Autodesk Inventor part; units mm, degrees
(part 2 of 13)
  line L395 (2.337, 43.029) -> (2.4628, 43.029)
  arc A395 (2.4628, 43.029) -> (2.4628, 43.155) centre (2.4628, 43.092) ccw
  line L396 (2.4628, 43.155) -> (2.337, 43.155)
  arc A396 (2.337, 43.155) -> (2.337, 43.029) centre (2.337, 43.092) ccw
  line L397 (3.263, 43.029) -> (17.121, 43.029)
  arc A397 (17.121, 43.029) -> (17.121, 43.155) centre (17.121, 43.092) ccw
  line L398 (17.121, 43.155) -> (3.263, 43.155)
  arc A398 (3.263, 43.155) -> (3.263, 43.029) centre (3.263, 43.092) ccw
  line L399 (1.0789, 43.155) -> (1.4109, 43.155)
  arc A399 (1.4109, 43.155) -> (1.4109, 43.281) centre (1.4109, 43.218) ccw
  line L400 (1.4109, 43.281) -> (1.0789, 43.281)
  arc A400 (1.0789, 43.281) -> (1.0789, 43.155) centre (1.0789, 43.218) ccw
  line L401 (2.337, 43.155) -> (2.4628, 43.155)
  arc A401 (2.4628, 43.155) -> (2.4628, 43.281) centre (2.4628, 43.218) ccw
  line L402 (2.4628, 43.281) -> (2.337, 43.281)
  arc A402 (2.337, 43.281) -> (2.337, 43.155) centre (2.337, 43.218) ccw
  line L403 (3.389, 43.155) -> (17.121, 43.155)
  arc A403 (17.121, 43.155) -> (17.121, 43.281) centre (17.121, 43.218) ccw
  line L404 (17.121, 43.281) -> (3.389, 43.281)
  arc A404 (3.389, 43.281) -> (3.389, 43.155) centre (3.389, 43.218) ccw
  line L405 (1.0789, 43.281) -> (1.3337, 43.281)
  arc A405 (1.3337, 43.281) -> (1.3337, 43.407) centre (1.3337, 43.344) ccw
  line L406 (1.3337, 43.407) -> (1.0789, 43.407)
  arc A406 (1.0789, 43.407) -> (1.0789, 43.281) centre (1.0789, 43.344) ccw
  line L407 (2.337, 43.281) -> (2.4628, 43.281)
  arc A407 (2.4628, 43.281) -> (2.4628, 43.407) centre (2.4628, 43.344) ccw
  line L408 (2.4628, 43.407) -> (2.337, 43.407)
  arc A408 (2.337, 43.407) -> (2.337, 43.281) centre (2.337, 43.344) ccw
  line L409 (3.4661, 43.281) -> (17.121, 43.281)
  arc A409 (17.121, 43.281) -> (17.121, 43.407) centre (17.121, 43.344) ccw
  line L410 (17.121, 43.407) -> (3.4661, 43.407)
  arc A410 (3.4661, 43.407) -> (3.4661, 43.281) centre (3.4661, 43.344) ccw
  line L411 (1.0789, 43.407) -> (1.2815, 43.407)
  arc A411 (1.2815, 43.407) -> (1.2815, 43.533) centre (1.2815, 43.47) ccw
  line L412 (1.2815, 43.533) -> (1.0789, 43.533)
  arc A412 (1.0789, 43.533) -> (1.0789, 43.407) centre (1.0789, 43.47) ccw
  line L413 (2.337, 43.407) -> (2.4628, 43.407)
  arc A413 (2.4628, 43.407) -> (2.4628, 43.533) centre (2.4628, 43.47) ccw
  line L414 (2.4628, 43.533) -> (2.337, 43.533)
  arc A414 (2.337, 43.533) -> (2.337, 43.407) centre (2.337, 43.47) ccw
  line L415 (3.5183, 43.407) -> (7.3627, 43.407)
  arc A415 (7.3627, 43.407) -> (7.3627, 43.533) centre (7.3627, 43.47) ccw
  line L416 (7.3627, 43.533) -> (3.5183, 43.533)
  arc A416 (3.5183, 43.533) -> (3.5183, 43.407) centre (3.5183, 43.47) ccw
  line L417 (8.0371, 43.407) -> (17.121, 43.407)
  arc A417 (17.121, 43.407) -> (17.121, 43.533) centre (17.121, 43.47) ccw
  line L418 (17.121, 43.533) -> (8.0371, 43.533)
  arc A418 (8.0371, 43.533) -> (8.0371, 43.407) centre (8.0371, 43.47) ccw
  line L419 (1.0789, 43.533) -> (1.2293, 43.533)
  arc A419 (1.2293, 43.533) -> (1.2293, 43.659) centre (1.2293, 43.596) ccw
  line L420 (1.2293, 43.659) -> (1.0789, 43.659)
  arc A420 (1.0789, 43.659) -> (1.0789, 43.533) centre (1.0789, 43.596) ccw
  line L421 (2.337, 43.533) -> (2.4628, 43.533)
  arc A421 (2.4628, 43.533) -> (2.4628, 43.659) centre (2.4628, 43.596) ccw
  line L422 (2.4628, 43.659) -> (2.337, 43.659)
  arc A422 (2.337, 43.659) -> (2.337, 43.533) centre (2.337, 43.596) ccw
  line L423 (3.5705, 43.533) -> (7.0585, 43.533)
  arc A423 (7.0585, 43.533) -> (7.0585, 43.659) centre (7.0585, 43.596) ccw
  line L424 (7.0585, 43.659) -> (3.5705, 43.659)
  arc A424 (3.5705, 43.659) -> (3.5705, 43.533) centre (3.5705, 43.596) ccw
  line L425 (8.3413, 43.533) -> (17.121, 43.533)
  arc A425 (17.121, 43.533) -> (17.121, 43.659) centre (17.121, 43.596) ccw
  line L426 (17.121, 43.659) -> (8.3413, 43.659)
  arc A426 (8.3413, 43.659) -> (8.3413, 43.533) centre (8.3413, 43.596) ccw
  line L427 (1.0789, 43.659) -> (1.183, 43.659)
  arc A427 (1.183, 43.659) -> (1.183, 43.785) centre (1.183, 43.722) ccw
  line L428 (1.183, 43.785) -> (1.0789, 43.785)
  arc A428 (1.0789, 43.785) -> (1.0789, 43.659) centre (1.0789, 43.722) ccw
  line L429 (2.337, 43.659) -> (2.4628, 43.659)
  arc A429 (2.4628, 43.659) -> (2.4628, 43.785) centre (2.4628, 43.722) ccw
  line L430 (2.4628, 43.785) -> (2.337, 43.785)
  arc A430 (2.337, 43.785) -> (2.337, 43.659) centre (2.337, 43.722) ccw
  line L431 (3.6169, 43.659) -> (6.8884, 43.659)
  arc A431 (6.8884, 43.659) -> (6.8884, 43.785) centre (6.8884, 43.722) ccw
  line L432 (6.8884, 43.785) -> (3.6169, 43.785)
  arc A432 (3.6169, 43.785) -> (3.6169, 43.659) centre (3.6169, 43.722) ccw
  line L433 (8.5115, 43.659) -> (17.121, 43.659)
  arc A433 (17.121, 43.659) -> (17.121, 43.785) centre (17.121, 43.722) ccw
  line L434 (17.121, 43.785) -> (8.5115, 43.785)
  arc A434 (8.5115, 43.785) -> (8.5115, 43.659) centre (8.5115, 43.722) ccw
  line L435 (1.0789, 43.785) -> (1.183, 43.785)
  arc A435 (1.183, 43.785) -> (1.183, 43.911) centre (1.183, 43.848) ccw
  line L436 (1.183, 43.911) -> (1.0789, 43.911)
  arc A436 (1.0789, 43.911) -> (1.0789, 43.785) centre (1.0789, 43.848) ccw
  line L437 (2.337, 43.785) -> (2.4628, 43.785)
  arc A437 (2.4628, 43.785) -> (2.4628, 43.911) centre (2.4628, 43.848) ccw
  line L438 (2.4628, 43.911) -> (2.337, 43.911)
  arc A438 (2.337, 43.911) -> (2.337, 43.785) centre (2.337, 43.848) ccw
  line L439 (3.6169, 43.785) -> (6.7624, 43.785)
  arc A439 (6.7624, 43.785) -> (6.7624, 43.911) centre (6.7624, 43.848) ccw
  line L440 (6.7624, 43.911) -> (3.6169, 43.911)
  arc A440 (3.6169, 43.911) -> (3.6169, 43.785) centre (3.6169, 43.848) ccw
  line L441 (8.6375, 43.785) -> (17.121, 43.785)
  arc A441 (17.121, 43.785) -> (17.121, 43.911) centre (17.121, 43.848) ccw
  line L442 (17.121, 43.911) -> (8.6375, 43.911)
  arc A442 (8.6375, 43.911) -> (8.6375, 43.785) centre (8.6375, 43.848) ccw
  line L443 (1.0789, 43.911) -> (2.3365, 43.911)
  arc A443 (2.3365, 43.911) -> (2.3365, 44.037) centre (2.3365, 43.974) ccw
  line L444 (2.3365, 44.037) -> (1.0789, 44.037)
  arc A444 (1.0789, 44.037) -> (1.0789, 43.911) centre (1.0789, 43.974) ccw
  line L445 (2.4634, 43.911) -> (6.6364, 43.911)
  arc A445 (6.6364, 43.911) -> (6.6364, 44.037) centre (6.6364, 43.974) ccw
  line L446 (6.6364, 44.037) -> (2.4634, 44.037)
  arc A446 (2.4634, 44.037) -> (2.4634, 43.911) centre (2.4634, 43.974) ccw
  line L447 (8.7635, 43.911) -> (17.121, 43.911)
  arc A447 (17.121, 43.911) -> (17.121, 44.037) centre (17.121, 43.974) ccw
  line L448 (17.121, 44.037) -> (8.7635, 44.037)
  arc A448 (8.7635, 44.037) -> (8.7635, 43.911) centre (8.7635, 43.974) ccw
  line L449 (1.0789, 44.037) -> (1.183, 44.037)
  arc A449 (1.183, 44.037) -> (1.183, 44.163) centre (1.183, 44.1) ccw
  line L450 (1.183, 44.163) -> (1.0789, 44.163)
  arc A450 (1.0789, 44.163) -> (1.0789, 44.037) centre (1.0789, 44.1) ccw
  line L451 (2.337, 44.037) -> (2.4628, 44.037)
  arc A451 (2.4628, 44.037) -> (2.4628, 44.163) centre (2.4628, 44.1) ccw
  line L452 (2.4628, 44.163) -> (2.337, 44.163)
  arc A452 (2.337, 44.163) -> (2.337, 44.037) centre (2.337, 44.1) ccw
  line L453 (3.6169, 44.037) -> (6.5788, 44.037)
  arc A453 (6.5788, 44.037) -> (6.5788, 44.163) centre (6.5788, 44.1) ccw
  line L454 (6.5788, 44.163) -> (3.6169, 44.163)
  arc A454 (3.6169, 44.163) -> (3.6169, 44.037) centre (3.6169, 44.1) ccw
  line L455 (8.821, 44.037) -> (17.121, 44.037)
  arc A455 (17.121, 44.037) -> (17.121, 44.163) centre (17.121, 44.1) ccw
  line L456 (17.121, 44.163) -> (8.821, 44.163)
  arc A456 (8.821, 44.163) -> (8.821, 44.037) centre (8.821, 44.1) ccw
  line L457 (1.0789, 44.163) -> (1.1971, 44.163)
  arc A457 (1.1971, 44.163) -> (1.1971, 44.289) centre (1.1971, 44.226) ccw
  line L458 (1.1971, 44.289) -> (1.0789, 44.289)
  arc A458 (1.0789, 44.289) -> (1.0789, 44.163) centre (1.0789, 44.226) ccw
  line L459 (2.337, 44.163) -> (2.4628, 44.163)
  arc A459 (2.4628, 44.163) -> (2.4628, 44.289) centre (2.4628, 44.226) ccw
  line L460 (2.4628, 44.289) -> (2.337, 44.289)
  arc A460 (2.337, 44.289) -> (2.337, 44.163) centre (2.337, 44.226) ccw
  line L461 (3.6029, 44.163) -> (6.5266, 44.163)
  arc A461 (6.5266, 44.163) -> (6.5266, 44.289) centre (6.5266, 44.226) ccw
  line L462 (6.5266, 44.289) -> (3.6029, 44.289)
  arc A462 (3.6029, 44.289) -> (3.6029, 44.163) centre (3.6029, 44.226) ccw
  line L463 (8.8732, 44.163) -> (17.121, 44.163)
  arc A463 (17.121, 44.163) -> (17.121, 44.289) centre (17.121, 44.226) ccw
  line L464 (17.121, 44.289) -> (8.8732, 44.289)
  arc A464 (8.8732, 44.289) -> (8.8732, 44.163) centre (8.8732, 44.226) ccw
  line L465 (1.0789, 44.289) -> (1.2493, 44.289)
  arc A465 (1.2493, 44.289) -> (1.2493, 44.415) centre (1.2493, 44.352) ccw
  line L466 (1.2493, 44.415) -> (1.0789, 44.415)
  arc A466 (1.0789, 44.415) -> (1.0789, 44.289) centre (1.0789, 44.352) ccw
  line L467 (2.337, 44.289) -> (2.4628, 44.289)
  arc A467 (2.4628, 44.289) -> (2.4628, 44.415) centre (2.4628, 44.352) ccw
  line L468 (2.4628, 44.415) -> (2.337, 44.415)
  arc A468 (2.337, 44.415) -> (2.337, 44.289) centre (2.337, 44.352) ccw
  line L469 (3.5507, 44.289) -> (6.4744, 44.289)
  arc A469 (6.4744, 44.289) -> (6.4744, 44.415) centre (6.4744, 44.352) ccw
  line L470 (6.4744, 44.415) -> (3.5507, 44.415)
  arc A470 (3.5507, 44.415) -> (3.5507, 44.289) centre (3.5507, 44.352) ccw
  line L471 (8.9254, 44.289) -> (17.121, 44.289)
  arc A471 (17.121, 44.289) -> (17.121, 44.415) centre (17.121, 44.352) ccw
  line L472 (17.121, 44.415) -> (8.9254, 44.415)
  arc A472 (8.9254, 44.415) -> (8.9254, 44.289) centre (8.9254, 44.352) ccw
  line L473 (1.0789, 44.415) -> (1.3015, 44.415)
  arc A473 (1.3015, 44.415) -> (1.3015, 44.541) centre (1.3015, 44.478) ccw
  line L474 (1.3015, 44.541) -> (1.0789, 44.541)
  arc A474 (1.0789, 44.541) -> (1.0789, 44.415) centre (1.0789, 44.478) ccw
  line L475 (2.337, 44.415) -> (2.4628, 44.415)
  arc A475 (2.4628, 44.415) -> (2.4628, 44.541) centre (2.4628, 44.478) ccw
  line L476 (2.4628, 44.541) -> (2.337, 44.541)
  arc A476 (2.337, 44.541) -> (2.337, 44.415) centre (2.337, 44.478) ccw
  line L477 (3.4985, 44.415) -> (6.4346, 44.415)
  arc A477 (6.4346, 44.415) -> (6.4346, 44.541) centre (6.4346, 44.478) ccw
  line L478 (6.4346, 44.541) -> (3.4985, 44.541)
  arc A478 (3.4985, 44.541) -> (3.4985, 44.415) centre (3.4985, 44.478) ccw
  line L479 (8.9653, 44.415) -> (17.121, 44.415)
  arc A479 (17.121, 44.415) -> (17.121, 44.541) centre (17.121, 44.478) ccw
  line L480 (17.121, 44.541) -> (8.9653, 44.541)
  arc A480 (8.9653, 44.541) -> (8.9653, 44.415) centre (8.9653, 44.478) ccw
  line L481 (1.0789, 44.541) -> (1.3537, 44.541)
  arc A481 (1.3537, 44.541) -> (1.3537, 44.667) centre (1.3537, 44.604) ccw
  line L482 (1.3537, 44.667) -> (1.0789, 44.667)
  arc A482 (1.0789, 44.667) -> (1.0789, 44.541) centre (1.0789, 44.604) ccw
  line L483 (2.337, 44.541) -> (2.4628, 44.541)
  arc A483 (2.4628, 44.541) -> (2.4628, 44.667) centre (2.4628, 44.604) ccw
  line L484 (2.4628, 44.667) -> (2.337, 44.667)
  arc A484 (2.337, 44.667) -> (2.337, 44.541) centre (2.337, 44.604) ccw
  line L485 (3.4463, 44.541) -> (6.4346, 44.541)
  arc A485 (6.4346, 44.541) -> (6.4346, 44.667) centre (6.4346, 44.604) ccw
  line L486 (6.4346, 44.667) -> (3.4463, 44.667)
  arc A486 (3.4463, 44.667) -> (3.4463, 44.541) centre (3.4463, 44.604) ccw
  line L487 (8.9653, 44.541) -> (17.121, 44.541)
  arc A487 (17.121, 44.541) -> (17.121, 44.667) centre (17.121, 44.604) ccw
  line L488 (17.121, 44.667) -> (8.9653, 44.667)
  arc A488 (8.9653, 44.667) -> (8.9653, 44.541) centre (8.9653, 44.604) ccw
  line L489 (1.0789, 44.667) -> (1.459, 44.667)
  arc A489 (1.459, 44.667) -> (1.459, 44.793) centre (1.459, 44.73) ccw
  line L490 (1.459, 44.793) -> (1.0789, 44.793)
  arc A490 (1.0789, 44.793) -> (1.0789, 44.667) centre (1.0789, 44.73) ccw
  line L491 (2.337, 44.667) -> (2.4628, 44.667)
  arc A491 (2.4628, 44.667) -> (2.4628, 44.793) centre (2.4628, 44.73) ccw
  line L492 (2.4628, 44.793) -> (2.337, 44.793)
  arc A492 (2.337, 44.793) -> (2.337, 44.667) centre (2.337, 44.73) ccw
  line L493 (3.3409, 44.667) -> (6.4346, 44.667)
  arc A493 (6.4346, 44.667) -> (6.4346, 44.793) centre (6.4346, 44.73) ccw
  line L494 (6.4346, 44.793) -> (3.3409, 44.793)
  arc A494 (3.3409, 44.793) -> (3.3409, 44.667) centre (3.3409, 44.73) ccw
  line L495 (8.9653, 44.667) -> (17.121, 44.667)
  arc A495 (17.121, 44.667) -> (17.121, 44.793) centre (17.121, 44.73) ccw
  line L496 (17.121, 44.793) -> (8.9653, 44.793)
  arc A496 (8.9653, 44.793) -> (8.9653, 44.667) centre (8.9653, 44.73) ccw
  line L497 (1.0789, 44.793) -> (1.585, 44.793)
  arc A497 (1.585, 44.793) -> (1.585, 44.919) centre (1.585, 44.856) ccw
  line L498 (1.585, 44.919) -> (1.0789, 44.919)
  arc A498 (1.0789, 44.919) -> (1.0789, 44.793) centre (1.0789, 44.856) ccw
  line L499 (2.337, 44.793) -> (2.4628, 44.793)
  arc A499 (2.4628, 44.793) -> (2.4628, 44.919) centre (2.4628, 44.856) ccw
  line L500 (2.4628, 44.919) -> (2.337, 44.919)
  arc A500 (2.337, 44.919) -> (2.337, 44.793) centre (2.337, 44.856) ccw
  line L501 (3.2149, 44.793) -> (6.4346, 44.793)
  arc A501 (6.4346, 44.793) -> (6.4346, 44.919) centre (6.4346, 44.856) ccw
  line L502 (6.4346, 44.919) -> (3.2149, 44.919)
  arc A502 (3.2149, 44.919) -> (3.2149, 44.793) centre (3.2149, 44.856) ccw
  line L503 (8.9653, 44.793) -> (17.121, 44.793)
  arc A503 (17.121, 44.793) -> (17.121, 44.919) centre (17.121, 44.856) ccw
  line L504 (17.121, 44.919) -> (8.9653, 44.919)
  arc A504 (8.9653, 44.919) -> (8.9653, 44.793) centre (8.9653, 44.856) ccw
  line L505 (1.0789, 44.919) -> (1.7116, 44.919)
  arc A505 (1.7116, 44.919) -> (1.7116, 45.045) centre (1.7116, 44.982) ccw
  line L506 (1.7116, 45.045) -> (1.0789, 45.045)
  arc A506 (1.0789, 45.045) -> (1.0789, 44.919) centre (1.0789, 44.982) ccw
  line L507 (2.337, 44.919) -> (2.4628, 44.919)
  arc A507 (2.4628, 44.919) -> (2.4628, 45.045) centre (2.4628, 44.982) ccw
  line L508 (2.4628, 45.045) -> (2.337, 45.045)
  arc A508 (2.337, 45.045) -> (2.337, 44.919) centre (2.337, 44.982) ccw
  line L509 (3.0884, 44.919) -> (6.4472, 44.919)
  arc A509 (6.4472, 44.919) -> (6.4472, 45.045) centre (6.4472, 44.982) ccw
  line L510 (6.4472, 45.045) -> (3.0884, 45.045)
  arc A510 (3.0884, 45.045) -> (3.0884, 44.919) centre (3.0884, 44.982) ccw
  line L511 (8.9528, 44.919) -> (17.121, 44.919)
  arc A511 (17.121, 44.919) -> (17.121, 45.045) centre (17.121, 44.982) ccw
  line L512 (17.121, 45.045) -> (8.9528, 45.045)
  arc A512 (8.9528, 45.045) -> (8.9528, 44.919) centre (8.9528, 44.982) ccw
  line L513 (1.0789, 45.045) -> (2.0157, 45.045)
  arc A513 (2.0157, 45.045) -> (2.0157, 45.171) centre (2.0157, 45.108) ccw
  line L514 (2.0157, 45.171) -> (1.0789, 45.171)
  arc A514 (1.0789, 45.171) -> (1.0789, 45.045) centre (1.0789, 45.108) ccw
  line L515 (2.337, 45.045) -> (2.4628, 45.045)
  arc A515 (2.4628, 45.045) -> (2.4628, 45.171) centre (2.4628, 45.108) ccw
  line L516 (2.4628, 45.171) -> (2.337, 45.171)
  arc A516 (2.337, 45.171) -> (2.337, 45.045) centre (2.337, 45.108) ccw
  line L517 (2.7843, 45.045) -> (6.4994, 45.045)
  arc A517 (6.4994, 45.045) -> (6.4994, 45.171) centre (6.4994, 45.108) ccw
  line L518 (6.4994, 45.171) -> (2.7843, 45.171)
  arc A518 (2.7843, 45.171) -> (2.7843, 45.045) centre (2.7843, 45.108) ccw
  line L519 (8.9006, 45.045) -> (17.121, 45.045)
  arc A519 (17.121, 45.045) -> (17.121, 45.171) centre (17.121, 45.108) ccw
  line L520 (17.121, 45.171) -> (8.9006, 45.171)
  arc A520 (8.9006, 45.171) -> (8.9006, 45.045) centre (8.9006, 45.108) ccw
  line L521 (1.0789, 45.171) -> (6.5516, 45.171)
  arc A521 (6.5516, 45.171) -> (6.5516, 45.297) centre (6.5516, 45.234) ccw
  line L522 (6.5516, 45.297) -> (1.0789, 45.297)
  arc A522 (1.0789, 45.297) -> (1.0789, 45.171) centre (1.0789, 45.234) ccw
  line L523 (8.8484, 45.171) -> (17.121, 45.171)
  arc A523 (17.121, 45.171) -> (17.121, 45.297) centre (17.121, 45.234) ccw
  line L524 (17.121, 45.297) -> (8.8484, 45.297)
  arc A524 (8.8484, 45.297) -> (8.8484, 45.171) centre (8.8484, 45.234) ccw
  line L525 (1.0789, 45.297) -> (6.6038, 45.297)
  arc A525 (6.6038, 45.297) -> (6.6038, 45.423) centre (6.6038, 45.36) ccw
  line L526 (6.6038, 45.423) -> (1.0789, 45.423)
  arc A526 (1.0789, 45.423) -> (1.0789, 45.297) centre (1.0789, 45.36) ccw
  line L527 (8.7962, 45.297) -> (17.121, 45.297)
  arc A527 (17.121, 45.297) -> (17.121, 45.423) centre (17.121, 45.36) ccw
  line L528 (17.121, 45.423) -> (8.7962, 45.423)
  arc A528 (8.7962, 45.423) -> (8.7962, 45.297) centre (8.7962, 45.36) ccw
  line L529 (1.0789, 45.423) -> (6.6965, 45.423)
  arc A529 (6.6965, 45.423) -> (6.6965, 45.549) centre (6.6965, 45.486) ccw
  line L530 (6.6965, 45.549) -> (1.0789, 45.549)
  arc A530 (1.0789, 45.549) -> (1.0789, 45.423) centre (1.0789, 45.486) ccw
  line L531 (8.7034, 45.423) -> (17.121, 45.423)
  arc A531 (17.121, 45.423) -> (17.121, 45.549) centre (17.121, 45.486) ccw
  line L532 (17.121, 45.549) -> (8.7034, 45.549)
  arc A532 (8.7034, 45.549) -> (8.7034, 45.423) centre (8.7034, 45.486) ccw
  line L533 (1.0789, 45.549) -> (6.8225, 45.549)
  arc A533 (6.8225, 45.549) -> (6.8225, 45.675) centre (6.8225, 45.612) ccw
  line L534 (6.8225, 45.675) -> (1.0789, 45.675)
  arc A534 (1.0789, 45.675) -> (1.0789, 45.549) centre (1.0789, 45.612) ccw
  line L535 (8.5774, 45.549) -> (17.121, 45.549)
  arc A535 (17.121, 45.549) -> (17.121, 45.675) centre (17.121, 45.612) ccw
  line L536 (17.121, 45.675) -> (8.5774, 45.675)
  arc A536 (8.5774, 45.675) -> (8.5774, 45.549) centre (8.5774, 45.612) ccw
  line L537 (1.0789, 45.675) -> (6.9485, 45.675)
  arc A537 (6.9485, 45.675) -> (6.9485, 45.801) centre (6.9485, 45.738) ccw
  line L538 (6.9485, 45.801) -> (1.0789, 45.801)
  arc A538 (1.0789, 45.801) -> (1.0789, 45.675) centre (1.0789, 45.738) ccw
  line L539 (8.4514, 45.675) -> (17.121, 45.675)
  arc A539 (17.121, 45.675) -> (17.121, 45.801) centre (17.121, 45.738) ccw
  line L540 (17.121, 45.801) -> (8.4514, 45.801)
  arc A540 (8.4514, 45.801) -> (8.4514, 45.675) centre (8.4514, 45.738) ccw
  line L541 (1.0789, 45.801) -> (7.2037, 45.801)
  arc A541 (7.2037, 45.801) -> (7.2037, 45.927) centre (7.2037, 45.864) ccw
  line L542 (7.2037, 45.927) -> (1.0789, 45.927)
  arc A542 (1.0789, 45.927) -> (1.0789, 45.801) centre (1.0789, 45.864) ccw
  line L543 (8.1963, 45.801) -> (17.121, 45.801)
  arc A543 (17.121, 45.801) -> (17.121, 45.927) centre (17.121, 45.864) ccw
  line L544 (17.121, 45.927) -> (8.1963, 45.927)
  arc A544 (8.1963, 45.927) -> (8.1963, 45.801) centre (8.1963, 45.864) ccw
  line L545 (1.0789, 45.927) -> (17.121, 45.927)
  arc A545 (17.121, 45.927) -> (17.121, 46.053) centre (17.121, 45.99) ccw
  line L546 (17.121, 46.053) -> (1.0789, 46.053)
  arc A546 (1.0789, 46.053) -> (1.0789, 45.927) centre (1.0789, 45.99) ccw
  line L547 (1.0789, 46.053) -> (17.121, 46.053)
  arc A547 (17.121, 46.053) -> (17.121, 46.179) centre (17.121, 46.116) ccw
  line L548 (17.121, 46.179) -> (1.0789, 46.179)
  arc A548 (1.0789, 46.179) -> (1.0789, 46.053) centre (1.0789, 46.116) ccw
  line L549 (1.0789, 46.179) -> (17.121, 46.179)
  arc A549 (17.121, 46.179) -> (17.121, 46.305) centre (17.121, 46.242) ccw
  line L550 (17.121, 46.305) -> (1.0789, 46.305)
  arc A550 (1.0789, 46.305) -> (1.0789, 46.179) centre (1.0789, 46.242) ccw
  line L551 (1.0789, 46.305) -> (2.0974, 46.305)
  arc A551 (2.0974, 46.305) -> (2.0974, 46.431) centre (2.0974, 46.368) ccw
  line L552 (2.0974, 46.431) -> (1.0789, 46.431)
  arc A552 (1.0789, 46.431) -> (1.0789, 46.305) centre (1.0789, 46.368) ccw
  line L553 (2.7024, 46.305) -> (17.121, 46.305)
  arc A553 (17.121, 46.305) -> (17.121, 46.431) centre (17.121, 46.368) ccw
  line L554 (17.121, 46.431) -> (2.7024, 46.431)
  arc A554 (2.7024, 46.431) -> (2.7024, 46.305) centre (2.7024, 46.368) ccw
  line L555 (1.0789, 46.431) -> (1.7932, 46.431)
  arc A555 (1.7932, 46.431) -> (1.7932, 46.557) centre (1.7932, 46.494) ccw
  line L556 (1.7932, 46.557) -> (1.0789, 46.557)
  arc A556 (1.0789, 46.557) -> (1.0789, 46.431) centre (1.0789, 46.494) ccw
  line L557 (3.0066, 46.431) -> (17.121, 46.431)
  arc A557 (17.121, 46.431) -> (17.121, 46.557) centre (17.121, 46.494) ccw
  line L558 (17.121, 46.557) -> (3.0066, 46.557)
  arc A558 (3.0066, 46.557) -> (3.0066, 46.431) centre (3.0066, 46.494) ccw
  line L559 (1.0789, 46.557) -> (1.6525, 46.557)
  arc A559 (1.6525, 46.557) -> (1.6525, 46.683) centre (1.6525, 46.62) ccw
  line L560 (1.6525, 46.683) -> (1.0789, 46.683)
  arc A560 (1.0789, 46.683) -> (1.0789, 46.557) centre (1.0789, 46.62) ccw
  line L561 (3.1474, 46.557) -> (17.121, 46.557)
  arc A561 (17.121, 46.557) -> (17.121, 46.683) centre (17.121, 46.62) ccw
  line L562 (17.121, 46.683) -> (3.1474, 46.683)
  arc A562 (3.1474, 46.683) -> (3.1474, 46.557) centre (3.1474, 46.62) ccw
  line L563 (1.0789, 46.683) -> (1.5265, 46.683)
  arc A563 (1.5265, 46.683) -> (1.5265, 46.809) centre (1.5265, 46.746) ccw
  line L564 (1.5265, 46.809) -> (1.0789, 46.809)
  arc A564 (1.0789, 46.809) -> (1.0789, 46.683) centre (1.0789, 46.746) ccw
  line L565 (3.2734, 46.683) -> (17.121, 46.683)
  arc A565 (17.121, 46.683) -> (17.121, 46.809) centre (17.121, 46.746) ccw
  line L566 (17.121, 46.809) -> (3.2734, 46.809)
  arc A566 (3.2734, 46.809) -> (3.2734, 46.683) centre (3.2734, 46.746) ccw
  line L567 (1.0789, 46.809) -> (1.432, 46.809)
  arc A567 (1.432, 46.809) -> (1.432, 46.935) centre (1.432, 46.872) ccw
  line L568 (1.432, 46.935) -> (1.0789, 46.935)
  arc A568 (1.0789, 46.935) -> (1.0789, 46.809) centre (1.0789, 46.872) ccw
  line L569 (3.3678, 46.809) -> (17.121, 46.809)
  arc A569 (17.121, 46.809) -> (17.121, 46.935) centre (17.121, 46.872) ccw
  line L570 (17.121, 46.935) -> (3.3678, 46.935)
  arc A570 (3.3678, 46.935) -> (3.3678, 46.809) centre (3.3678, 46.872) ccw
  line L571 (1.0789, 46.935) -> (1.3798, 46.935)
  arc A571 (1.3798, 46.935) -> (1.3798, 47.061) centre (1.3798, 46.998) ccw
  line L572 (1.3798, 47.061) -> (1.0789, 47.061)
  arc A572 (1.0789, 47.061) -> (1.0789, 46.935) centre (1.0789, 46.998) ccw
  line L573 (3.42, 46.935) -> (17.121, 46.935)
  arc A573 (17.121, 46.935) -> (17.121, 47.061) centre (17.121, 46.998) ccw
  line L574 (17.121, 47.061) -> (3.42, 47.061)
  arc A574 (3.42, 47.061) -> (3.42, 46.935) centre (3.42, 46.998) ccw
  line L575 (1.0789, 47.061) -> (1.3277, 47.061)
  arc A575 (1.3277, 47.061) -> (1.3277, 47.187) centre (1.3277, 47.124) ccw
  line L576 (1.3277, 47.187) -> (1.0789, 47.187)
  arc A576 (1.0789, 47.187) -> (1.0789, 47.061) centre (1.0789, 47.124) ccw
  line L577 (3.4721, 47.061) -> (17.121, 47.061)
  arc A577 (17.121, 47.061) -> (17.121, 47.187) centre (17.121, 47.124) ccw
  line L578 (17.121, 47.187) -> (3.4721, 47.187)
  arc A578 (3.4721, 47.187) -> (3.4721, 47.061) centre (3.4721, 47.124) ccw
  line L579 (1.0789, 47.187) -> (1.2846, 47.187)
  arc A579 (1.2846, 47.187) -> (1.2846, 47.313) centre (1.2846, 47.25) ccw
  line L580 (1.2846, 47.313) -> (1.0789, 47.313)
  arc A580 (1.0789, 47.313) -> (1.0789, 47.187) centre (1.0789, 47.25) ccw
  line L581 (3.5153, 47.187) -> (17.121, 47.187)
  arc A581 (17.121, 47.187) -> (17.121, 47.313) centre (17.121, 47.25) ccw
  line L582 (17.121, 47.313) -> (3.5153, 47.313)
  arc A582 (3.5153, 47.313) -> (3.5153, 47.187) centre (3.5153, 47.25) ccw
  line L583 (1.0789, 47.313) -> (1.2846, 47.313)
  arc A583 (1.2846, 47.313) -> (1.2846, 47.439) centre (1.2846, 47.376) ccw
  line L584 (1.2846, 47.439) -> (1.0789, 47.439)
  arc A584 (1.0789, 47.439) -> (1.0789, 47.313) centre (1.0789, 47.376) ccw
  line L585 (3.5153, 47.313) -> (17.121, 47.313)
  arc A585 (17.121, 47.313) -> (17.121, 47.439) centre (17.121, 47.376) ccw
  line L586 (17.121, 47.439) -> (3.5153, 47.439)
  arc A586 (3.5153, 47.439) -> (3.5153, 47.313) centre (3.5153, 47.376) ccw
  line L587 (1.0789, 47.439) -> (1.2846, 47.439)
  arc A587 (1.2846, 47.439) -> (1.2846, 47.565) centre (1.2846, 47.502) ccw
  line L588 (1.2846, 47.565) -> (1.0789, 47.565)
  arc A588 (1.0789, 47.565) -> (1.0789, 47.439) centre (1.0789, 47.502) ccw
  line L589 (3.5153, 47.439) -> (17.121, 47.439)
  arc A589 (17.121, 47.439) -> (17.121, 47.565) centre (17.121, 47.502) ccw
  line L590 (17.121, 47.565) -> (3.5153, 47.565)
  arc A590 (3.5153, 47.565) -> (3.5153, 47.439) centre (3.5153, 47.502) ccw
  line L591 (1.0789, 47.565) -> (1.2846, 47.565)
  arc A591 (1.2846, 47.565) -> (1.2846, 47.691) centre (1.2846, 47.628) ccw
  line L592 (1.2846, 47.691) -> (1.0789, 47.691)
  arc A592 (1.0789, 47.691) -> (1.0789, 47.565) centre (1.0789, 47.628) ccw
  line L593 (3.5153, 47.565) -> (17.121, 47.565)
  arc A593 (17.121, 47.565) -> (17.121, 47.691) centre (17.121, 47.628) ccw
  line L594 (17.121, 47.691) -> (3.5153, 47.691)
  arc A594 (3.5153, 47.691) -> (3.5153, 47.565) centre (3.5153, 47.628) ccw
  line L595 (1.0789, 47.691) -> (1.3187, 47.691)
  arc A595 (1.3187, 47.691) -> (1.3187, 47.817) centre (1.3187, 47.754) ccw
  line L596 (1.3187, 47.817) -> (1.0789, 47.817)
  arc A596 (1.0789, 47.817) -> (1.0789, 47.691) centre (1.0789, 47.754) ccw
  line L597 (3.4813, 47.691) -> (17.121, 47.691)
  arc A597 (17.121, 47.691) -> (17.121, 47.817) centre (17.121, 47.754) ccw
  line L598 (17.121, 47.817) -> (3.4813, 47.817)
  arc A598 (3.4813, 47.817) -> (3.4813, 47.691) centre (3.4813, 47.754) ccw
  line L599 (1.0789, 47.817) -> (1.3709, 47.817)
  arc A599 (1.3709, 47.817) -> (1.3709, 47.943) centre (1.3709, 47.88) ccw
  line L600 (1.3709, 47.943) -> (1.0789, 47.943)
  arc A600 (1.0789, 47.943) -> (1.0789, 47.817) centre (1.0789, 47.88) ccw
  line L601 (3.4291, 47.817) -> (17.121, 47.817)
  arc A601 (17.121, 47.817) -> (17.121, 47.943) centre (17.121, 47.88) ccw
  line L602 (17.121, 47.943) -> (3.4291, 47.943)
  arc A602 (3.4291, 47.943) -> (3.4291, 47.817) centre (3.4291, 47.88) ccw
  line L603 (1.0789, 47.943) -> (1.4231, 47.943)
  arc A603 (1.4231, 47.943) -> (1.4231, 48.069) centre (1.4231, 48.006) ccw
  line L604 (1.4231, 48.069) -> (1.0789, 48.069)
  arc A604 (1.0789, 48.069) -> (1.0789, 47.943) centre (1.0789, 48.006) ccw
  line L605 (3.3769, 47.943) -> (17.121, 47.943)
  arc A605 (17.121, 47.943) -> (17.121, 48.069) centre (17.121, 48.006) ccw
  line L606 (17.121, 48.069) -> (3.3769, 48.069)
  arc A606 (3.3769, 48.069) -> (3.3769, 47.943) centre (3.3769, 48.006) ccw
  line L607 (1.0789, 48.069) -> (1.5046, 48.069)
  arc A607 (1.5046, 48.069) -> (1.5046, 48.195) centre (1.5046, 48.132) ccw
  line L608 (1.5046, 48.195) -> (1.0789, 48.195)
  arc A608 (1.0789, 48.195) -> (1.0789, 48.069) centre (1.0789, 48.132) ccw
  line L609 (3.2953, 48.069) -> (17.121, 48.069)
  arc A609 (17.121, 48.069) -> (17.121, 48.195) centre (17.121, 48.132) ccw
  line L610 (17.121, 48.195) -> (3.2953, 48.195)
  arc A610 (3.2953, 48.195) -> (3.2953, 48.069) centre (3.2953, 48.132) ccw
  line L611 (1.0789, 48.195) -> (1.6306, 48.195)
  arc A611 (1.6306, 48.195) -> (1.6306, 48.321) centre (1.6306, 48.258) ccw
  line L612 (1.6306, 48.321) -> (1.0789, 48.321)
  arc A612 (1.0789, 48.321) -> (1.0789, 48.195) centre (1.0789, 48.258) ccw
  line L613 (3.1693, 48.195) -> (17.121, 48.195)
  arc A613 (17.121, 48.195) -> (17.121, 48.321) centre (17.121, 48.258) ccw
  line L614 (17.121, 48.321) -> (3.1693, 48.321)
  arc A614 (3.1693, 48.321) -> (3.1693, 48.195) centre (3.1693, 48.258) ccw
  line L615 (1.0789, 48.321) -> (1.7566, 48.321)
  arc A615 (1.7566, 48.321) -> (1.7566, 48.447) centre (1.7566, 48.384) ccw
  line L616 (1.7566, 48.447) -> (1.0789, 48.447)
  arc A616 (1.0789, 48.447) -> (1.0789, 48.321) centre (1.0789, 48.384) ccw
  line L617 (3.0433, 48.321) -> (17.121, 48.321)
  arc A617 (17.121, 48.321) -> (17.121, 48.447) centre (17.121, 48.384) ccw
  line L618 (17.121, 48.447) -> (3.0433, 48.447)
  arc A618 (3.0433, 48.447) -> (3.0433, 48.321) centre (3.0433, 48.384) ccw
  line L619 (1.0789, 48.447) -> (2.0446, 48.447)
  arc A619 (2.0446, 48.447) -> (2.0446, 48.573) centre (2.0446, 48.51) ccw
  line L620 (2.0446, 48.573) -> (1.0789, 48.573)
  arc A620 (1.0789, 48.573) -> (1.0789, 48.447) centre (1.0789, 48.51) ccw
  line L621 (2.7554, 48.447) -> (7.1938, 48.447)
  arc A621 (7.1938, 48.447) -> (7.1938, 48.573) centre (7.1938, 48.51) ccw
  line L622 (7.1938, 48.573) -> (2.7554, 48.573)
  arc A622 (2.7554, 48.573) -> (2.7554, 48.447) centre (2.7554, 48.51) ccw
  line L623 (7.637, 48.447) -> (7.7628, 48.447)
  arc A623 (7.7628, 48.447) -> (7.7628, 48.573) centre (7.7628, 48.51) ccw
  line L624 (7.7628, 48.573) -> (7.637, 48.573)
  arc A624 (7.637, 48.573) -> (7.637, 48.447) centre (7.637, 48.51) ccw
  line L625 (8.206, 48.447) -> (17.121, 48.447)
  arc A625 (17.121, 48.447) -> (17.121, 48.573) centre (17.121, 48.51) ccw
  line L626 (17.121, 48.573) -> (8.206, 48.573)
  arc A626 (8.206, 48.573) -> (8.206, 48.447) centre (8.206, 48.51) ccw
  line L627 (1.0789, 48.573) -> (6.9107, 48.573)
  arc A627 (6.9107, 48.573) -> (6.9107, 48.699) centre (6.9107, 48.636) ccw
  line L628 (6.9107, 48.699) -> (1.0789, 48.699)
  arc A628 (1.0789, 48.699) -> (1.0789, 48.573) centre (1.0789, 48.636) ccw
  line L629 (7.637, 48.573) -> (7.7628, 48.573)
  arc A629 (7.7628, 48.573) -> (7.7628, 48.699) centre (7.7628, 48.636) ccw
  line L630 (7.7628, 48.699) -> (7.637, 48.699)
  arc A630 (7.637, 48.699) -> (7.637, 48.573) centre (7.637, 48.636) ccw
  line L631 (8.4892, 48.573) -> (17.121, 48.573)
  arc A631 (17.121, 48.573) -> (17.121, 48.699) centre (17.121, 48.636) ccw
  line L632 (17.121, 48.699) -> (8.4892, 48.699)
  arc A632 (8.4892, 48.699) -> (8.4892, 48.573) centre (8.4892, 48.636) ccw
  line L633 (1.0789, 48.699) -> (6.7847, 48.699)
  arc A633 (6.7847, 48.699) -> (6.7847, 48.825) centre (6.7847, 48.762) ccw
  line L634 (6.7847, 48.825) -> (1.0789, 48.825)
  arc A634 (1.0789, 48.825) -> (1.0789, 48.699) centre (1.0789, 48.762) ccw
  line L635 (7.637, 48.699) -> (7.7628, 48.699)
  arc A635 (7.7628, 48.699) -> (7.7628, 48.825) centre (7.7628, 48.762) ccw
  line L636 (7.7628, 48.825) -> (7.637, 48.825)
  arc A636 (7.637, 48.825) -> (7.637, 48.699) centre (7.637, 48.762) ccw
  line L637 (8.6152, 48.699) -> (17.121, 48.699)
  arc A637 (17.121, 48.699) -> (17.121, 48.825) centre (17.121, 48.762) ccw
  line L638 (17.121, 48.825) -> (8.6152, 48.825)
  arc A638 (8.6152, 48.825) -> (8.6152, 48.699) centre (8.6152, 48.762) ccw
  line L639 (1.0789, 48.825) -> (6.6587, 48.825)
  arc A639 (6.6587, 48.825) -> (6.6587, 48.951) centre (6.6587, 48.888) ccw
  line L640 (6.6587, 48.951) -> (1.0789, 48.951)
  arc A640 (1.0789, 48.951) -> (1.0789, 48.825) centre (1.0789, 48.888) ccw
  line L641 (7.637, 48.825) -> (7.7628, 48.825)
  arc A641 (7.7628, 48.825) -> (7.7628, 48.951) centre (7.7628, 48.888) ccw
  line L642 (7.7628, 48.951) -> (7.637, 48.951)
  arc A642 (7.637, 48.951) -> (7.637, 48.825) centre (7.637, 48.888) ccw
  line L643 (8.7412, 48.825) -> (17.121, 48.825)
  arc A643 (17.121, 48.825) -> (17.121, 48.951) centre (17.121, 48.888) ccw
  line L644 (17.121, 48.951) -> (8.7412, 48.951)
  arc A644 (8.7412, 48.951) -> (8.7412, 48.825) centre (8.7412, 48.888) ccw
  line L645 (1.0789, 48.951) -> (6.5376, 48.951)
  arc A645 (6.5376, 48.951) -> (6.5376, 49.077) centre (6.5376, 49.014) ccw
  line L646 (6.5376, 49.077) -> (1.0789, 49.077)
  arc A646 (1.0789, 49.077) -> (1.0789, 48.951) centre (1.0789, 49.014) ccw
  line L647 (7.637, 48.951) -> (7.7628, 48.951)
  arc A647 (7.7628, 48.951) -> (7.7628, 49.077) centre (7.7628, 49.014) ccw
  line L648 (7.7628, 49.077) -> (7.637, 49.077)
  arc A648 (7.637, 49.077) -> (7.637, 48.951) centre (7.637, 49.014) ccw
  line L649 (8.8622, 48.951) -> (17.121, 48.951)
  arc A649 (17.121, 48.951) -> (17.121, 49.077) centre (17.121, 49.014) ccw
  line L650 (17.121, 49.077) -> (8.8622, 49.077)
  arc A650 (8.8622, 49.077) -> (8.8622, 48.951) centre (8.8622, 49.014) ccw
  line L651 (1.0789, 49.077) -> (6.4854, 49.077)
  arc A651 (6.4854, 49.077) -> (6.4854, 49.203) centre (6.4854, 49.14) ccw
  line L652 (6.4854, 49.203) -> (1.0789, 49.203)
  arc A652 (1.0789, 49.203) -> (1.0789, 49.077) centre (1.0789, 49.14) ccw
  line L653 (7.637, 49.077) -> (7.7628, 49.077)
  arc A653 (7.7628, 49.077) -> (7.7628, 49.203) centre (7.7628, 49.14) ccw
  line L654 (7.7628, 49.203) -> (7.637, 49.203)
  arc A654 (7.637, 49.203) -> (7.637, 49.077) centre (7.637, 49.14) ccw
  line L655 (8.9144, 49.077) -> (17.121, 49.077)
  arc A655 (17.121, 49.077) -> (17.121, 49.203) centre (17.121, 49.14) ccw
  line L656 (17.121, 49.203) -> (8.9144, 49.203)
  arc A656 (8.9144, 49.203) -> (8.9144, 49.077) centre (8.9144, 49.14) ccw
  line L657 (1.0789, 49.203) -> (6.4332, 49.203)
  arc A657 (6.4332, 49.203) -> (6.4332, 49.329) centre (6.4332, 49.266) ccw
  line L658 (6.4332, 49.329) -> (1.0789, 49.329)
  arc A658 (1.0789, 49.329) -> (1.0789, 49.203) centre (1.0789, 49.266) ccw
  line L659 (7.637, 49.203) -> (7.7628, 49.203)
  arc A659 (7.7628, 49.203) -> (7.7628, 49.329) centre (7.7628, 49.266) ccw
  line L660 (7.7628, 49.329) -> (7.637, 49.329)
  arc A660 (7.637, 49.329) -> (7.637, 49.203) centre (7.637, 49.266) ccw
  line L661 (8.9666, 49.203) -> (17.121, 49.203)
  arc A661 (17.121, 49.203) -> (17.121, 49.329) centre (17.121, 49.266) ccw
  line L662 (17.121, 49.329) -> (8.9666, 49.329)
  arc A662 (8.9666, 49.329) -> (8.9666, 49.203) centre (8.9666, 49.266) ccw
  line L663 (1.0789, 49.329) -> (6.381, 49.329)
  arc A663 (6.381, 49.329) -> (6.381, 49.455) centre (6.381, 49.392) ccw
  line L664 (6.381, 49.455) -> (1.0789, 49.455)
  arc A664 (1.0789, 49.455) -> (1.0789, 49.329) centre (1.0789, 49.392) ccw
  line L665 (7.637, 49.329) -> (7.7628, 49.329)
  arc A665 (7.7628, 49.329) -> (7.7628, 49.455) centre (7.7628, 49.392) ccw
  line L666 (7.7628, 49.455) -> (7.637, 49.455)
  arc A666 (7.637, 49.455) -> (7.637, 49.329) centre (7.637, 49.392) ccw
  line L667 (9.0188, 49.329) -> (17.121, 49.329)
  arc A667 (17.121, 49.329) -> (17.121, 49.455) centre (17.121, 49.392) ccw
  line L668 (17.121, 49.455) -> (9.0188, 49.455)
  arc A668 (9.0188, 49.455) -> (9.0188, 49.329) centre (9.0188, 49.392) ccw
  line L669 (1.0789, 49.455) -> (6.333, 49.455)
  arc A669 (6.333, 49.455) -> (6.333, 49.581) centre (6.333, 49.518) ccw
  line L670 (6.333, 49.581) -> (1.0789, 49.581)
  arc A670 (1.0789, 49.581) -> (1.0789, 49.455) centre (1.0789, 49.518) ccw
  line L671 (7.637, 49.455) -> (7.7628, 49.455)
  arc A671 (7.7628, 49.455) -> (7.7628, 49.581) centre (7.7628, 49.518) ccw
  line L672 (7.7628, 49.581) -> (7.637, 49.581)
  arc A672 (7.637, 49.581) -> (7.637, 49.455) centre (7.637, 49.518) ccw
  line L673 (9.0669, 49.455) -> (17.121, 49.455)
  arc A673 (17.121, 49.455) -> (17.121, 49.581) centre (17.121, 49.518) ccw
  line L674 (17.121, 49.581) -> (9.0669, 49.581)
  arc A674 (9.0669, 49.581) -> (9.0669, 49.455) centre (9.0669, 49.518) ccw
  line L675 (1.0789, 49.581) -> (6.333, 49.581)
  arc A675 (6.333, 49.581) -> (6.333, 49.707) centre (6.333, 49.644) ccw
  line L676 (6.333, 49.707) -> (1.0789, 49.707)
  arc A676 (1.0789, 49.707) -> (1.0789, 49.581) centre (1.0789, 49.644) ccw
  line L677 (7.637, 49.581) -> (7.7628, 49.581)
  arc A677 (7.7628, 49.581) -> (7.7628, 49.707) centre (7.7628, 49.644) ccw
  line L678 (7.7628, 49.707) -> (7.637, 49.707)
  arc A678 (7.637, 49.707) -> (7.637, 49.581) centre (7.637, 49.644) ccw
  line L679 (9.0669, 49.581) -> (17.121, 49.581)
  arc A679 (17.121, 49.581) -> (17.121, 49.707) centre (17.121, 49.644) ccw
  line L680 (17.121, 49.707) -> (9.0669, 49.707)
  arc A680 (9.0669, 49.707) -> (9.0669, 49.581) centre (9.0669, 49.644) ccw
  line L681 (1.0789, 49.707) -> (2.0685, 49.707)
  arc A681 (2.0685, 49.707) -> (2.0685, 49.833) centre (2.0685, 49.77) ccw
  line L682 (2.0685, 49.833) -> (1.0789, 49.833)
  arc A682 (1.0789, 49.833) -> (1.0789, 49.707) centre (1.0789, 49.77) ccw
  line L683 (2.337, 49.707) -> (2.4628, 49.707)
  arc A683 (2.4628, 49.707) -> (2.4628, 49.833) centre (2.4628, 49.77) ccw
  line L684 (2.4628, 49.833) -> (2.337, 49.833)
  arc A684 (2.337, 49.833) -> (2.337, 49.707) centre (2.337, 49.77) ccw
  line L685 (2.7313, 49.707) -> (7.6365, 49.707)
  arc A685 (7.6365, 49.707) -> (7.6365, 49.833) centre (7.6365, 49.77) ccw
  line L686 (7.6365, 49.833) -> (2.7313, 49.833)
  arc A686 (2.7313, 49.833) -> (2.7313, 49.707) centre (2.7313, 49.77) ccw
  line L687 (7.7634, 49.707) -> (17.121, 49.707)
  arc A687 (17.121, 49.707) -> (17.121, 49.833) centre (17.121, 49.77) ccw
  line L688 (17.121, 49.833) -> (7.7634, 49.833)
  arc A688 (7.7634, 49.833) -> (7.7634, 49.707) centre (7.7634, 49.77) ccw
  arc A689 (1.7644, 49.833) -> (1.7644, 49.959) centre (1.7644, 49.896) ccw
  line L689 (1.7644, 49.959) -> (1.0789, 49.959)
  arc A690 (1.0789, 49.959) -> (1.0789, 49.833) centre (1.0789, 49.896) ccw
  line L690 (2.337, 49.833) -> (2.4628, 49.833)
  arc A691 (2.4628, 49.833) -> (2.4628, 49.959) centre (2.4628, 49.896) ccw
  line L691 (2.4628, 49.959) -> (2.337, 49.959)
  arc A692 (2.337, 49.959) -> (2.337, 49.833) centre (2.337, 49.896) ccw
  line L692 (3.0354, 49.833) -> (6.333, 49.833)
  arc A693 (6.333, 49.833) -> (6.333, 49.959) centre (6.333, 49.896) ccw
  line L693 (6.333, 49.959) -> (3.0354, 49.959)
  arc A694 (3.0354, 49.959) -> (3.0354, 49.833) centre (3.0354, 49.896) ccw
  line L694 (7.637, 49.833) -> (7.7628, 49.833)
  arc A695 (7.7628, 49.833) -> (7.7628, 49.959) centre (7.7628, 49.896) ccw
  line L695 (7.7628, 49.959) -> (7.637, 49.959)
  arc A696 (7.637, 49.959) -> (7.637, 49.833) centre (7.637, 49.896) ccw
  line L696 (9.0669, 49.833) -> (17.121, 49.833)
  arc A697 (17.121, 49.833) -> (17.121, 49.959) centre (17.121, 49.896) ccw
  line L697 (17.121, 49.959) -> (9.0669, 49.959)
  arc A698 (9.0669, 49.959) -> (9.0669, 49.833) centre (9.0669, 49.896) ccw
  line L698 (1.0789, 49.959) -> (1.6069, 49.959)
  arc A699 (1.6069, 49.959) -> (1.6069, 50.085) centre (1.6069, 50.022) ccw
  line L699 (1.6069, 50.085) -> (1.0789, 50.085)
  arc A700 (1.0789, 50.085) -> (1.0789, 49.959) centre (1.0789, 50.022) ccw
  line L700 (2.337, 49.959) -> (2.4628, 49.959)
  arc A701 (2.4628, 49.959) -> (2.4628, 50.085) centre (2.4628, 50.022) ccw
  line L701 (2.4628, 50.085) -> (2.337, 50.085)
  arc A702 (2.337, 50.085) -> (2.337, 49.959) centre (2.337, 50.022) ccw
  line L702 (3.193, 49.959) -> (6.333, 49.959)
  arc A703 (6.333, 49.959) -> (6.333, 50.085) centre (6.333, 50.022) ccw
  line L703 (6.333, 50.085) -> (3.193, 50.085)
  arc A704 (3.193, 50.085) -> (3.193, 49.959) centre (3.193, 50.022) ccw
  line L704 (7.637, 49.959) -> (7.7628, 49.959)
  arc A705 (7.7628, 49.959) -> (7.7628, 50.085) centre (7.7628, 50.022) ccw
  line L705 (7.7628, 50.085) -> (7.637, 50.085)
  arc A706 (7.637, 50.085) -> (7.637, 49.959) centre (7.637, 50.022) ccw
  line L706 (9.0669, 49.959) -> (17.121, 49.959)
  arc A707 (17.121, 49.959) -> (17.121, 50.085) centre (17.121, 50.022) ccw
  line L707 (17.121, 50.085) -> (9.0669, 50.085)
  arc A708 (9.0669, 50.085) -> (9.0669, 49.959) centre (9.0669, 50.022) ccw
  line L708 (1.0789, 50.085) -> (1.4809, 50.085)
  arc A709 (1.4809, 50.085) -> (1.4809, 50.211) centre (1.4809, 50.148) ccw
  line L709 (1.4809, 50.211) -> (1.0789, 50.211)
  arc A710 (1.0789, 50.211) -> (1.0789, 50.085) centre (1.0789, 50.148) ccw
  line L710 (2.337, 50.085) -> (2.4628, 50.085)
  arc A711 (2.4628, 50.085) -> (2.4628, 50.211) centre (2.4628, 50.148) ccw
  line L711 (2.4628, 50.211) -> (2.337, 50.211)
  arc A712 (2.337, 50.211) -> (2.337, 50.085) centre (2.337, 50.148) ccw
  line L712 (3.319, 50.085) -> (6.3729, 50.085)
  arc A713 (6.3729, 50.085) -> (6.3729, 50.211) centre (6.3729, 50.148) ccw
  line L713 (6.3729, 50.211) -> (3.319, 50.211)
  arc A714 (3.319, 50.211) -> (3.319, 50.085) centre (3.319, 50.148) ccw
  line L714 (7.637, 50.085) -> (7.7628, 50.085)
  arc A715 (7.7628, 50.085) -> (7.7628, 50.211) centre (7.7628, 50.148) ccw
  line L715 (7.7628, 50.211) -> (7.637, 50.211)
  arc A716 (7.637, 50.211) -> (7.637, 50.085) centre (7.637, 50.148) ccw
  line L716 (9.0271, 50.085) -> (17.121, 50.085)
  arc A717 (17.121, 50.085) -> (17.121, 50.211) centre (17.121, 50.148) ccw
  line L717 (17.121, 50.211) -> (9.0271, 50.211)
  arc A718 (9.0271, 50.211) -> (9.0271, 50.085) centre (9.0271, 50.148) ccw
  line L718 (1.0789, 50.211) -> (1.3627, 50.211)
  arc A719 (1.3627, 50.211) -> (1.3627, 50.337) centre (1.3627, 50.274) ccw
  line L719 (1.3627, 50.337) -> (1.0789, 50.337)
  arc A720 (1.0789, 50.337) -> (1.0789, 50.211) centre (1.0789, 50.274) ccw
  line L720 (2.337, 50.211) -> (2.4628, 50.211)
  arc A721 (2.4628, 50.211) -> (2.4628, 50.337) centre (2.4628, 50.274) ccw
  line L721 (2.4628, 50.337) -> (2.337, 50.337)
  arc A722 (2.337, 50.337) -> (2.337, 50.211) centre (2.337, 50.274) ccw
  line L722 (3.4371, 50.211) -> (6.425, 50.211)
  arc A723 (6.425, 50.211) -> (6.425, 50.337) centre (6.425, 50.274) ccw
  line L723 (6.425, 50.337) -> (3.4371, 50.337)
  arc A724 (3.4371, 50.337) -> (3.4371, 50.211) centre (3.4371, 50.274) ccw
  line L724 (7.637, 50.211) -> (7.7628, 50.211)
  arc A725 (7.7628, 50.211) -> (7.7628, 50.337) centre (7.7628, 50.274) ccw
  line L725 (7.7628, 50.337) -> (7.637, 50.337)
  arc A726 (7.637, 50.337) -> (7.637, 50.211) centre (7.637, 50.274) ccw
  line L726 (8.975, 50.211) -> (17.121, 50.211)
  arc A727 (17.121, 50.211) -> (17.121, 50.337) centre (17.121, 50.274) ccw
  line L727 (17.121, 50.337) -> (8.975, 50.337)
  arc A728 (8.975, 50.337) -> (8.975, 50.211) centre (8.975, 50.274) ccw
  line L728 (1.0789, 50.337) -> (1.3105, 50.337)
  arc A729 (1.3105, 50.337) -> (1.3105, 50.463) centre (1.3105, 50.4) ccw
  line L729 (1.3105, 50.463) -> (1.0789, 50.463)
  arc A730 (1.0789, 50.463) -> (1.0789, 50.337) centre (1.0789, 50.4) ccw
  line L730 (2.337, 50.337) -> (2.4628, 50.337)
  arc A731 (2.4628, 50.337) -> (2.4628, 50.463) centre (2.4628, 50.4) ccw
  line L731 (2.4628, 50.463) -> (2.337, 50.463)
  arc A732 (2.337, 50.463) -> (2.337, 50.337) centre (2.337, 50.4) ccw
  line L732 (3.4893, 50.337) -> (6.4772, 50.337)
  arc A733 (6.4772, 50.337) -> (6.4772, 50.463) centre (6.4772, 50.4) ccw
  line L733 (6.4772, 50.463) -> (3.4893, 50.463)
  arc A734 (3.4893, 50.463) -> (3.4893, 50.337) centre (3.4893, 50.4) ccw
  line L734 (7.637, 50.337) -> (7.7628, 50.337)
  arc A735 (7.7628, 50.337) -> (7.7628, 50.463) centre (7.7628, 50.4) ccw
  line L735 (7.7628, 50.463) -> (7.637, 50.463)
  arc A736 (7.637, 50.463) -> (7.637, 50.337) centre (7.637, 50.4) ccw
  line L736 (8.9228, 50.337) -> (17.121, 50.337)
  arc A737 (17.121, 50.337) -> (17.121, 50.463) centre (17.121, 50.4) ccw
  line L737 (17.121, 50.463) -> (8.9228, 50.463)
  arc A738 (8.9228, 50.463) -> (8.9228, 50.337) centre (8.9228, 50.4) ccw
  line L738 (1.0789, 50.463) -> (1.2583, 50.463)
  arc A739 (1.2583, 50.463) -> (1.2583, 50.589) centre (1.2583, 50.526) ccw
  line L739 (1.2583, 50.589) -> (1.0789, 50.589)
  arc A740 (1.0789, 50.589) -> (1.0789, 50.463) centre (1.0789, 50.526) ccw
  line L740 (2.337, 50.463) -> (2.4628, 50.463)
  arc A741 (2.4628, 50.463) -> (2.4628, 50.589) centre (2.4628, 50.526) ccw
  line L741 (2.4628, 50.589) -> (2.337, 50.589)
  arc A742 (2.337, 50.589) -> (2.337, 50.463) centre (2.337, 50.526) ccw
  line L742 (3.5415, 50.463) -> (6.5294, 50.463)
  arc A743 (6.5294, 50.463) -> (6.5294, 50.589) centre (6.5294, 50.526) ccw
  line L743 (6.5294, 50.589) -> (3.5415, 50.589)
  arc A744 (3.5415, 50.589) -> (3.5415, 50.463) centre (3.5415, 50.526) ccw
  line L744 (7.637, 50.463) -> (7.7628, 50.463)
  arc A745 (7.7628, 50.463) -> (7.7628, 50.589) centre (7.7628, 50.526) ccw
  line L745 (7.7628, 50.589) -> (7.637, 50.589)
  arc A746 (7.637, 50.589) -> (7.637, 50.463) centre (7.637, 50.526) ccw
  line L746 (8.8706, 50.463) -> (17.121, 50.463)
  arc A747 (17.121, 50.463) -> (17.121, 50.589) centre (17.121, 50.526) ccw
  line L747 (17.121, 50.589) -> (8.8706, 50.589)
  arc A748 (8.8706, 50.589) -> (8.8706, 50.463) centre (8.8706, 50.526) ccw
  line L748 (1.0789, 50.589) -> (1.2061, 50.589)
  arc A749 (1.2061, 50.589) -> (1.2061, 50.715) centre (1.2061, 50.652) ccw
  line L749 (1.2061, 50.715) -> (1.0789, 50.715)
  arc A750 (1.0789, 50.715) -> (1.0789, 50.589) centre (1.0789, 50.652) ccw
  line L750 (2.337, 50.589) -> (2.4628, 50.589)
  arc A751 (2.4628, 50.589) -> (2.4628, 50.715) centre (2.4628, 50.652) ccw
  line L751 (2.4628, 50.715) -> (2.337, 50.715)
  arc A752 (2.337, 50.715) -> (2.337, 50.589) centre (2.337, 50.652) ccw
  line L752 (3.5937, 50.589) -> (6.6388, 50.589)
  arc A753 (6.6388, 50.589) -> (6.6388, 50.715) centre (6.6388, 50.652) ccw
  line L753 (6.6388, 50.715) -> (3.5937, 50.715)
  arc A754 (3.5937, 50.715) -> (3.5937, 50.589) centre (3.5937, 50.652) ccw
  line L754 (7.637, 50.589) -> (7.7628, 50.589)
  arc A755 (7.7628, 50.589) -> (7.7628, 50.715) centre (7.7628, 50.652) ccw
  line L755 (7.7628, 50.715) -> (7.637, 50.715)
  arc A756 (7.637, 50.715) -> (7.637, 50.589) centre (7.637, 50.652) ccw
  line L756 (8.7611, 50.589) -> (17.121, 50.589)
  arc A757 (17.121, 50.589) -> (17.121, 50.715) centre (17.121, 50.652) ccw
  line L757 (17.121, 50.715) -> (8.7611, 50.715)
  arc A758 (8.7611, 50.715) -> (8.7611, 50.589) centre (8.7611, 50.652) ccw
  line L758 (1.0789, 50.715) -> (1.183, 50.715)
  arc A759 (1.183, 50.715) -> (1.183, 50.841) centre (1.183, 50.778) ccw
  line L759 (1.183, 50.841) -> (1.0789, 50.841)
  arc A760 (1.0789, 50.841) -> (1.0789, 50.715) centre (1.0789, 50.778) ccw
  line L760 (2.337, 50.715) -> (2.4628, 50.715)
  arc A761 (2.4628, 50.715) -> (2.4628, 50.841) centre (2.4628, 50.778) ccw
  line L761 (2.4628, 50.841) -> (2.337, 50.841)
  arc A762 (2.337, 50.841) -> (2.337, 50.715) centre (2.337, 50.778) ccw
  line L762 (3.6169, 50.715) -> (6.7648, 50.715)
  arc A763 (6.7648, 50.715) -> (6.7648, 50.841) centre (6.7648, 50.778) ccw
  line L763 (6.7648, 50.841) -> (3.6169, 50.841)
  arc A764 (3.6169, 50.841) -> (3.6169, 50.715) centre (3.6169, 50.778) ccw
  line L764 (7.637, 50.715) -> (7.7628, 50.715)
  arc A765 (7.7628, 50.715) -> (7.7628, 50.841) centre (7.7628, 50.778) ccw
  line L765 (7.7628, 50.841) -> (7.637, 50.841)
  arc A766 (7.637, 50.841) -> (7.637, 50.715) centre (7.637, 50.778) ccw
  line L766 (8.6351, 50.715) -> (17.121, 50.715)
  arc A767 (17.121, 50.715) -> (17.121, 50.841) centre (17.121, 50.778) ccw
  line L767 (17.121, 50.841) -> (8.6351, 50.841)
  arc A768 (8.6351, 50.841) -> (8.6351, 50.715) centre (8.6351, 50.778) ccw
  line L768 (1.0789, 50.841) -> (2.3365, 50.841)
  arc A769 (2.3365, 50.841) -> (2.3365, 50.967) centre (2.3365, 50.904) ccw
  line L769 (2.3365, 50.967) -> (1.0789, 50.967)
  arc A770 (1.0789, 50.967) -> (1.0789, 50.841) centre (1.0789, 50.904) ccw
  line L770 (2.4634, 50.841) -> (6.8908, 50.841)
  arc A771 (6.8908, 50.841) -> (6.8908, 50.967) centre (6.8908, 50.904) ccw
  line L771 (6.8908, 50.967) -> (2.4634, 50.967)
  arc A772 (2.4634, 50.967) -> (2.4634, 50.841) centre (2.4634, 50.904) ccw
  line L772 (7.637, 50.841) -> (7.7628, 50.841)
  arc A773 (7.7628, 50.841) -> (7.7628, 50.967) centre (7.7628, 50.904) ccw
  line L773 (7.7628, 50.967) -> (7.637, 50.967)
  arc A774 (7.637, 50.967) -> (7.637, 50.841) centre (7.637, 50.904) ccw
  line L774 (8.5091, 50.841) -> (17.121, 50.841)
  arc A775 (17.121, 50.841) -> (17.121, 50.967) centre (17.121, 50.904) ccw
  line L775 (17.121, 50.967) -> (8.5091, 50.967)
  arc A776 (8.5091, 50.967) -> (8.5091, 50.841) centre (8.5091, 50.904) ccw
  line L776 (1.0789, 50.967) -> (1.183, 50.967)
  arc A777 (1.183, 50.967) -> (1.183, 51.093) centre (1.183, 51.03) ccw
  line L777 (1.183, 51.093) -> (1.0789, 51.093)
  arc A778 (1.0789, 51.093) -> (1.0789, 50.967) centre (1.0789, 51.03) ccw
  line L778 (2.337, 50.967) -> (2.4628, 50.967)
  arc A779 (2.4628, 50.967) -> (2.4628, 51.093) centre (2.4628, 51.03) ccw
  line L779 (2.4628, 51.093) -> (2.337, 51.093)
  arc A780 (2.337, 51.093) -> (2.337, 50.967) centre (2.337, 51.03) ccw
  line L780 (3.6169, 50.967) -> (7.1458, 50.967)
  arc A781 (7.1458, 50.967) -> (7.1458, 51.093) centre (7.1458, 51.03) ccw
  line L781 (7.1458, 51.093) -> (3.6169, 51.093)
  arc A782 (3.6169, 51.093) -> (3.6169, 50.967) centre (3.6169, 51.03) ccw
  line L782 (7.637, 50.967) -> (7.7628, 50.967)
  arc A783 (7.7628, 50.967) -> (7.7628, 51.093) centre (7.7628, 51.03) ccw
  line L783 (7.7628, 51.093) -> (7.637, 51.093)
  arc A784 (7.637, 51.093) -> (7.637, 50.967) centre (7.637, 51.03) ccw
  line L784 (8.2542, 50.967) -> (17.121, 50.967)
  arc A785 (17.121, 50.967) -> (17.121, 51.093) centre (17.121, 51.03) ccw
  line L785 (17.121, 51.093) -> (8.2542, 51.093)
  arc A786 (8.2542, 51.093) -> (8.2542, 50.967) centre (8.2542, 51.03) ccw
  line L786 (1.0789, 51.093) -> (1.183, 51.093)
  arc A787 (1.183, 51.093) -> (1.183, 51.219) centre (1.183, 51.156) ccw
  line L787 (1.183, 51.219) -> (1.0789, 51.219)
  arc A788 (1.0789, 51.219) -> (1.0789, 51.093) centre (1.0789, 51.156) ccw
  line L788 (2.337, 51.093) -> (2.4628, 51.093)
  arc A789 (2.4628, 51.093) -> (2.4628, 51.219) centre (2.4628, 51.156) ccw
  line L789 (2.4628, 51.219) -> (2.337, 51.219)
  arc A790 (2.337, 51.219) -> (2.337, 51.093) centre (2.337, 51.156) ccw
  line L790 (3.6169, 51.093) -> (17.121, 51.093)
  arc A791 (17.121, 51.093) -> (17.121, 51.219) centre (17.121, 51.156) ccw
  line L791 (17.121, 51.219) -> (3.6169, 51.219)
  arc A792 (3.6169, 51.219) -> (3.6169, 51.093) centre (3.6169, 51.156) ccw
  line L792 (1.0789, 51.219) -> (1.2203, 51.219)
  arc A793 (1.2203, 51.219) -> (1.2203, 51.345) centre (1.2203, 51.282) ccw
  line L793 (1.2203, 51.345) -> (1.0789, 51.345)
  arc A794 (1.0789, 51.345) -> (1.0789, 51.219) centre (1.0789, 51.282) ccw
  line L794 (2.337, 51.219) -> (2.4628, 51.219)
  arc A795 (2.4628, 51.219) -> (2.4628, 51.345) centre (2.4628, 51.282) ccw
  arc A796 (17.121, 2.835) -> (17.121, 2.961) centre (17.121, 2.898) ccw
  line L795 (2.4628, 51.345) -> (2.337, 51.345)
  arc A797 (2.337, 51.345) -> (2.337, 51.219) centre (2.337, 51.282) ccw
  line L796 (3.5797, 51.219) -> (17.121, 51.219)